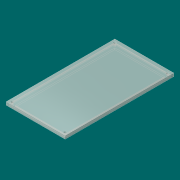
# Autodesk Inventor part: topBottom
Saved by Autodesk Inventor 2016 (Build 200138000, 138)
## iProperties
Created: 2015-10-13
Part Number: topBottom
Material: PC/ABS Plastic
Document SubType Name: Modeling
Designer: Sawaiz
Density: 0.357273 g/cm^3
Appearance: Clear
Author: Sawaiz
Autodesk Inventor part; units mm, degrees
ref_plane "YZ Plane" through (0, 0, 0) normal (1, 0, 0) x (0, 1, 0)
ref_plane "XZ Plane" through (0, 0, 0) normal (0, 1, 0) x (-1, 0, 0)
ref_plane "XY Plane" through (0, 0, 0) normal (0, 0, 1) x (1, 0, 0)
sketch "Sketch1" plane through (0, 0, 0) normal (0, 0, 1) x (1, 0, 0)
  line L0 (-111.125, -60.325) -> (111.125, -60.325)
  line L1 (111.125, -60.325) -> (111.125, 60.325)
  line L2 (111.125, 60.325) -> (-111.125, 60.325)
  line L3 (-111.125, 60.325) -> (-111.125, -60.325)
  line L4 (-111.125, -60.325) -> (111.125, 60.325) construction
  line L5 (111.125, -60.325) -> (-111.125, 60.325) construction
  point P0 (0, 0)
  dimension "d0" = 222.25
  dimension "d1" = 120.65
  constraints: 12 end point, 2 midpoint, 2 parallel, 1 horizontal, 1 perpendicular
  measures "d0" distance of L2.end L1.end
  measures "d1" distance of L1.end L0.end
extrude "Extrusion1" add sketch "Sketch1" along normal blind 9.525
sketch "Sketch12" plane through (0, 0, 9.525) normal (0, 0, 1) x (1, 0, 0)
  line L0 (-111.125, -60.325) -> (111.125, -60.325) projected
  line L1 (111.125, -60.325) -> (111.125, 60.325) projected
  line L2 (111.125, 60.325) -> (-111.125, 60.325) projected
  line L3 (-111.125, 60.325) -> (-111.125, -60.325) projected
  line L4 (104.775, -53.975) -> (-104.775, -53.975)
  line L5 (-104.775, -53.975) -> (-104.775, 53.975)
  line L6 (-104.775, 53.975) -> (104.775, 53.975)
  line L7 (104.775, 53.975) -> (104.775, -53.975)
  point P0 (0, 0)
  dimension "d87" = 6.35
  constraints: 8 end point, 4 coincident, 3 other
  measures "d87" distance between parallel lines of L0 L4
hole "Hole6" at (104.775, -53.975, 9.525) at (-104.775, -53.975, 9.525) at (-104.775, 53.975, 9.525) at (104.775, 53.975, 9.525) direction (0, 0, -1) diameter 3.264 end through all countersink diameter 5.715 countersink angle 82 clearance for "Flat Head Machine Screw (82)" size "#4" standard "Ansi Unified Screw Threads"
sketch "Sketch13" plane through (0, 0, 0) normal (0, 0, -1) x (-1, 0, 0)
  circle A0 centre (104.775, 53.975) radius 1.632 projected
  circle A1 centre (-104.775, -53.975) radius 1.632 projected
  circle A2 centre (104.775, -53.975) radius 1.632 projected
  circle A3 centre (-104.775, 53.975) radius 1.632 projected
  line L0 (111.125, -60.325) -> (-111.125, -60.325) projected
  line L1 (111.125, 60.325) -> (111.125, -60.325) projected
  line L2 (-111.125, 60.325) -> (111.125, 60.325) projected
  line L3 (-111.125, -60.325) -> (-111.125, 60.325) projected
  line L4 (-101.6, 50.8) -> (101.6, 50.8)
  line L5 (101.6, 50.8) -> (101.6, -50.8)
  line L6 (101.6, -50.8) -> (-101.6, -50.8)
  line L7 (-101.6, -50.8) -> (-101.6, 50.8)
  point P0 (0, 0)
  dimension "d95" = 9.525
  constraints: 8 end point, 3 other
  measures "d95" distance between parallel lines of L3 L7
extrude "Extrusion6" cut sketch "Sketch13" against normal blind 3.175
sketch "Sketch14" plane through (0, 0, 3.175) normal (0, 0, -1) x (-1, 0, 0)
  line L0 (-101.6, 50.8) -> (-101.6, -50.8) projected
  line L1 (101.6, 50.8) -> (-101.6, 50.8) projected
  line L2 (101.6, -50.8) -> (101.6, 50.8) projected
  line L3 (-101.6, -50.8) -> (101.6, -50.8) projected
  circle A0 centre (-104.775, 53.975) radius 1.632 projected
  circle A1 centre (104.775, -53.975) radius 1.632 projected
  circle A2 centre (-104.775, -53.975) radius 1.632 projected
  circle A3 centre (104.775, 53.975) radius 1.632 projected
  line L4 (111.125, -60.325) -> (-111.125, -60.325) projected
  line L5 (111.125, 60.325) -> (111.125, -60.325) projected
  line L6 (-111.125, 60.325) -> (111.125, 60.325) projected
  line L7 (-111.125, -60.325) -> (-111.125, 60.325) projected
  line L8 (-101.6, 50.8) -> (-101.6, -50.8) projected
  line L9 (-101.6, -50.8) -> (101.6, -50.8) projected
  line L10 (101.6, -50.8) -> (101.6, 50.8) projected
  line L11 (101.6, 50.8) -> (-101.6, 50.8) projected
  line L12 (-105.1179, 58.7375) -> (105.1179, 58.7375)
  line L13 (109.5375, 54.3179) -> (109.5375, -54.3179)
  line L14 (105.1179, -58.7375) -> (-105.1179, -58.7375)
  line L15 (-109.5375, -54.3179) -> (-109.5375, 54.3179)
  line L16 (-105.1179, 56.5277) -> (105.1179, 56.5277)
  line L17 (107.3277, 54.3179) -> (107.3277, -54.3179)
  line L18 (105.1179, -56.5277) -> (-105.1179, -56.5277)
  line L19 (-107.3277, -54.3179) -> (-107.3277, 54.3179)
  arc A4 (-107.3277, -54.3179) -> (-105.1179, -56.5277) centre (-105.1179, -54.3179) ccw
  arc A5 (-105.1179, 56.5277) -> (-107.3277, 54.3179) centre (-105.1179, 54.3179) ccw
  arc A6 (107.3277, 54.3179) -> (105.1179, 56.5277) centre (105.1179, 54.3179) ccw
  arc A7 (105.1179, -56.5277) -> (107.3277, -54.3179) centre (105.1179, -54.3179) ccw
  arc A8 (-109.5375, -54.3179) -> (-105.1179, -58.7375) centre (-105.1179, -54.3179) ccw
  arc A9 (-105.1179, 58.7375) -> (-109.5375, 54.3179) centre (-105.1179, 54.3179) ccw
  arc A10 (109.5375, 54.3179) -> (105.1179, 58.7375) centre (105.1179, 54.3179) ccw
  arc A11 (105.1179, -58.7375) -> (109.5375, -54.3179) centre (105.1179, -54.3179) ccw
  point P0 (0, 0)
  dimension "d101" = 1.5875
  dimension "d102" = 3.7973
  dimension "d103" = 2.2098
  dimension "d104" = 4.4196
  constraints: 16 end point, 16 point on circle, 16 tangent, 8 centre point, 6 equal radius, 6 other
  measures "d101" distance between parallel lines of L7 L15
  measures "d102" distance between parallel lines of L7 L19
  measures "d103" radius of A4
  measures "d104" radius of A8
extrude "Extrusion7" cut sketch "Sketch14" against normal blind 1.1684 contours L12 A10 L13 A11 L14 A8 L15 A9
equation "\"d0\" = depth + 2 * frameAcrylicThickness"
equation "\"d1\" = width + 2 * frameAcrylicThickness"
equation "\"d2\" = frameAcrylicThickness"
equation "\"d95\" = frameAcrylicThickness"
equation "\"acrylicThickness\" = 9.525"
equation "\"width\" = 101.6"
equation "\"depth\" = 203.2"
equation "\"oRingWidth\" = 1.5875"
equation "\"mirrorGroove\" = 19.05"
equation "\"mirrorGrooveMill\" = 3.175"
equation "\"height\" = 101.6"
equation "\"mirrorAngle\" = 5deg"
equation "\"detectorWidth\" = 52"
equation "\"detectorHeight\" = 52"
equation "\"mirrorThickness\" = 3.175"
equation "\"fresnelThickness\" = 0.1"
equation "\"focalLength\" = 76.2"
equation "\"ior\" = 1.49"
equation "\"centerThickness\" = 1.524"
equation "\"fresnelAngle\" = 90deg"
equation "\"fresnelEffectiveDiameter\" = 76.2"
equation "\"mirrorSuppourtWidth\" = 38.1"
equation "\"backGrooveBit\" = 4.8006"
equation "\"sensorHolderWidth\" = 88.9"
equation "\"sensorHolderHeight\" = 88.9"
equation "\"sensorHolderSensorHeight\" = 53.975"
equation "\"sensorHolderSensorWidth\" = 53.975"
equation "\"sensorHolderORingID\" = 203.2"
equation "\"sensorHolderFlushORingID\" = 304.8"
equation "\"frontBackORingID\" = 419.1"
equation "\"backMirrorGroove\" = 6.35"
equation "\"fresnelChamfer\" = 6.35"
equation "\"fresnelMirrorChamfer\" = 6.35"
equation "\"detectorOpeningHeight\" = 76.2"
equation "\"detectorOpeningWidth\" = 76.2"
equation "\"sensorHolderDepth\" = 19.05"
equation "\"frameAcrylicThickness\" = 9.525"
equation "\"internalAcrylicThicnkess\" = 6.35"
equation "\"aerogelHeight\" = 101.6"
equation "\"aerogelWidth\" = 101.6"
equation "\"internalAcrylicThickness\" = 6.35"
body "Solid1"
